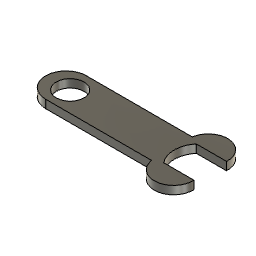
Exercise16 v1 (Autodesk Fusion 360 design; units mm, degrees)
Autodesk Fusion 360 part; units mm, degrees
sketch "Sketch2" plane through (0, 0, 0) normal (0, 0, 1) x (1, 0, 0)
  circle A0 centre (-70, 0) radius 17
  arc A1 (65, 20) -> (65, -20) centre (89.1778, 0) ccw
  line L0 (65, -20) -> (102, -20)
  line L1 (65, 19.9864) -> (102.1, 19.9864)
  line L2 (102.1, 19.9864) -> (102.1, -20)
  line L3 (102.1, -20) -> (65, -20)
  arc A2 (102.1, 19.9864) -> (55, 25) centre (78.4273, 21.3408) ccw
  arc A3 (55, -25) -> (102.1, -20) centre (78.427, -21.3413) ccw
  line L4 (55, 25) -> (-75, 25)
  line L5 (-75, 25) -> (-75, -25)
  line L6 (-75, -25) -> (55, -25)
  arc A4 (-75, 25) -> (-75, -25) centre (-75, 0) ccw
  point P0 (100, -20)
  point P1 (100, 20)
  point P2 (57.8, 0.0068)
  point P3 (55, 25)
  point P4 (55, -25)
  dimension "d3" = 34
  constraint coincident P2 A1
  constraint horizontal L1
  constraint perpendicular L0 L2
  constraint perpendicular L2 L3
  constraint coincident P3 A2.end
  constraint coincident P4 A3.start
  constraint horizontal L4
  constraint perpendicular L4 L5
  constraint perpendicular L5 L6
  constraint tangent L6 A4
  measures "d3" diameter of A0
sketch "Sketch3" plane through (0, 0, 0) normal (0, 0, 1) x (1, 0, 0)
  line L0 (65, 20) -> (102.1, 20)
  line L1 (102.1, 20) -> (102.1, -20)
  line L2 (102.1, -20) -> (65, -20)
  line L3 (65, -20) -> (65, 20)
  line L4 (65, 20) -> (65, -20)
  arc A0 (65, 20) -> (65, -20) centre (89.1778, 0) ccw
  constraint horizontal L0
  constraint vertical L1
  constraint horizontal L2
  constraint vertical L3
extrude "Extrude1" add sketch "Sketch2" along normal blind 10 contours A0 L2 A2 A3 L4 L5 L6 | A0 L5 A4
extrude "Extrude2" cut sketch "Sketch3" along normal blind 10
